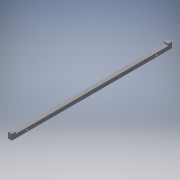
# Autodesk Inventor part: Support GuideRail
Saved by Autodesk Inventor 2016 (Build 200138000, 138)
## iProperties
Created: 2016-04-12
Part Number: Support GuideRail
Material: Generic
Document SubType Name: Modeling
Designer: aoben3
Density: 1 g/cm^3
Appearance: Default
Author: aoben3
Autodesk Inventor part; units mm, degrees
ref_plane "YZ Plane" through (0, 0, 0) normal (1, 0, 0) x (0, 1, 0)
ref_plane "XZ Plane" through (0, 0, 0) normal (0, 1, 0) x (-1, 0, 0)
ref_plane "XY Plane" through (0, 0, 0) normal (0, 0, 1) x (1, 0, 0)
sketch "Sketch1" plane through (0, 0, 0) normal (1, 0, 0) x (0, 1, 0)
  line L0 (3.3442, 266.7) -> (6.35, 266.7)
  line L1 (6.35, 266.7) -> (6.35, 254)
  line L2 (6.35, 254) -> (0, 254)
  line L3 (0, 254) -> (0, 0)
  line L4 (0, 0) -> (-12.7, 0) construction
  line L5 (-12.7, 0) -> (-12.7, 190.5)
  line L6 (-12.7, 215.9) -> (-12.7, 266.7)
  line L7 (3.3442, 266.7) -> (-12.7, 266.7)
  line L8 (3.3442, -266.7) -> (6.35, -266.7)
  line L9 (6.35, -266.7) -> (6.35, -254)
  line L10 (6.35, -254) -> (0, -254)
  line L11 (0, -254) -> (0, 0)
  line L12 (-12.7, 0) -> (-12.7, -190.5)
  line L13 (-12.7, -215.9) -> (-12.7, -266.7)
  line L14 (3.3442, -266.7) -> (-12.7, -266.7)
  line L15 (-12.7, 215.9) -> (-12.7, 190.5)
  line L16 (-12.7, -190.5) -> (-12.7, -215.9)
  dimension "d1" = 12.7
  dimension "d3" = 6.35
  dimension "d4" = 254
  dimension "d5" = 12.7
  constraints: 34 end point, 7 symmetric about line, 6 point on line, 5 perpendicular, 1 collinear, 1 horizontal, 1 parallel, 1 vertical
  measures "d1" distance of L3.end L4.end
  measures "d3" distance of L1.end L2.end
  measures "d4" distance between parallel lines of L4 L2
  measures "d5" distance of L0.end L1.end
extrude "Extrusion1" add sketch "Sketch1" along normal blind 12.7
sketch "Sketch4" plane through (12.7, 0, 0) normal (1, 0, 0) x (0, 0, -1)
  circle A0 centre (-215.9, -6.35) radius 2.921
  line L0 (-266.7, 6.35) -> (-266.7, -12.7) projected
  line L1 (254, 0) -> (-254, 0) projected
  point P0 (0, 0)
  dimension "d32" = 5.842
  dimension "d33" = 50.8
  dimension "d34" = 6.35
  constraints: 1 centre point
  measures "d32" diameter of A0
  measures "d33" distance from line of A0.centre L0
  measures "d34" distance from line of A0.centre L1
hole "Hole3" at (12.7, -6.35, 215.9) direction (-1, 0, 0) diameter 5.842 end through all
mirror "Mirror3" about plane through (0, 0, 0) normal (0, 0, 1) of "Hole3"
body "Solid1"
